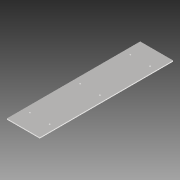
# Autodesk Inventor part: 4104_Aluminum Box Divider_V1
Saved by Autodesk Inventor 2020 (Build 240168000, 168)
## iProperties
Created: 2020-09-13
Part Number: 4104_Aluminum Box Divider_V1
Material: Aluminum 6061
Document SubType Name: Modeling
Designer: Eli Mattingly
Density: 2.7 g/cm^3
Appearance: Aluminum - Flat
Author: Eli Mattingly
Autodesk Inventor part; units mm, degrees
ref_plane "YZ Plane" through (0, 0, 0) normal (1, 0, 0) x (0, 1, 0)
ref_plane "XZ Plane" through (0, 0, 0) normal (0, 1, 0) x (-1, 0, 0)
ref_plane "XY Plane" through (0, 0, 0) normal (0, 0, 1) x (1, 0, 0)
sketch "Sketch1" plane through (0, 0, 0) normal (0, 0, 1) x (1, 0, 0)
  line L0 (-50, 1.5) -> (50, 1.5)
  line L1 (50, 1.5) -> (50, -1.5)
  line L2 (50, -1.5) -> (-50, -1.5)
  line L3 (-50, -1.5) -> (-50, 1.5)
  line L4 (-50, 1.5) -> (50, -1.5) construction
  line L5 (50, 1.5) -> (-50, -1.5) construction
  point P0 (0, 0)
  dimension "d0" = 100
  dimension "d1" = 3
  constraints: 12 end point, 2 midpoint, 2 parallel, 1 horizontal, 1 perpendicular
  measures "d0" distance of L1.end L2.end
  measures "d1" distance of L0.end L1.end
extrude "Extrusion1" add sketch "Sketch1" along normal mid plane 405
sketch "Sketch2" plane through (-50, -1.5, 202.5) normal (0, -1, 0) x (1, 0, 0)
  line L0 (0, 0) -> (100, 0) projected
  line L1 (0, -405) -> (0, 0) projected
  line L2 (100, -405) -> (0, -405) projected
  line L3 (100, 0) -> (0, 0) projected
  line L4 (20, 0) -> (20, -405)
  point P0 (50, -202.5)
  point P1 (20, -202.5)
  point P2 (20, -50)
  point P3 (20, -355)
  dimension "d4" = 20
  dimension "d5" = 50
  dimension "d6" = 50
  constraints: 4 point on line, 2 end point, 1 midpoint, 1 vertical
  measures "d4" distance between parallel lines of L1 L4
  measures "d5" distance from line of L2 point (20, -355)
  measures "d6" distance from line of L0 point (20, -50)
hole "Hole1" at (-30, -1.5, 0) at (-30, -1.5, 152.5) at (-30, -1.5, -152.5) direction (0, 1, 0) diameter 4 end through all
mirror "Mirror1" about plane through (0, 0, 0) normal (1, 0, 0) of "Hole1"
body "Solid1"
